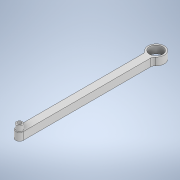
# Autodesk Inventor part: eslabon2
Saved by Autodesk Inventor 2021 (Build 250183000, 183)
## iProperties
Created: 2022-10-24
Part Number: eslabon2
Material: Genérico
Document SubType Name: Modeling
Designer: ivanm
Density: 1 g/cm^3
Appearance: Valor por defecto
Author: ivanm
Autodesk Inventor part; units mm, degrees
ref_plane "YZ Plane" through (0, 0, 0) normal (1, 0, 0) x (0, 1, 0)
ref_plane "XZ Plane" through (0, 0, 0) normal (0, 1, 0) x (-1, 0, 0)
ref_plane "XY Plane" through (0, 0, 0) normal (0, 0, 1) x (1, 0, 0)
sketch "Boceto2" plane through (0, 0, 0) normal (0, 1, 0) x (-1, 0, 0)
  arc A0 (5, 0) -> (-5, 0) centre (0, 0) ccw
  arc A1 (1.2, 2.1932) -> (1.2, -2.1932) centre (0, 0) ccw
  line L0 (1.2, 2.1932) -> (1.2, -2.1932)
  line L1 (0, 0) -> (0, -180)
  circle A2 centre (0, -180) radius 8.75
  arc A3 (-6.8254, -171.6948) -> (6.8254, -171.6948) centre (0, -180) ccw
  line L2 (5, 0) -> (5, -167.8319)
  line L3 (-5, 0) -> (-5, -167.8319)
  arc A4 (-6.8254, -171.6948) -> (-5, -167.8319) centre (-10, -167.8319) ccw
  arc A5 (5, -167.8319) -> (6.8254, -171.6948) centre (10, -167.8319) ccw
  point P0 (-5, -170.4836)
  point P1 (5, -170.4836)
  dimension "d13" = 10
  dimension "d14" = 5
  dimension "d15" = 1.2
  dimension "d16" = 180
  dimension "d17" = 17.5
  dimension "d18" = 2
  dimension "d19" = 5
  constraints: 12 point on circle, 8 end point, 6 centre point, 6 tangent, 4 coincident, 3 vertical, 2 point on line, 1 equal radius, 1 parallel
  measures "d13" diameter of A0
  measures "d14" diameter of A1
  measures "d15" distance from line of point (0, 0) L0
  measures "d16" distance of L1.start L1.end
  measures "d17" diameter of A2
  measures "d18" radial gap between concentric circles of A3 A2
  measures "d19" radius of A4
extrude "Extrusión2" add sketch "Boceto2" along normal blind 10
sketch "Boceto3" plane through (0, 10, 0) normal (0, 1, 0) x (1, 0, 0)
  circle A0 centre (0, 0) radius 4
  circle A1 centre (0, 0) radius 2.5
  dimension "d22" = 8
  constraints: 2 centre point, 2 coincident
  measures "d22" diameter of A0
extrude "Extrusión3" add sketch "Boceto3" along normal blind 7
